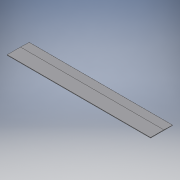
# Autodesk Inventor part: test_base
Saved by Autodesk Inventor 2018.1 (Build 221171000, 171)
## iProperties
Created: 2017-11-02
Part Number: test_base
Material: 一般
Document SubType Name: Modeling
Designer: kuwano
Density: 1 g/cm^3
Appearance: 既定
Author: kuwano
Autodesk Inventor part; units mm, degrees
ref_plane "XZ Plane" through (0, 0, 0) normal (0, 1, 0) x (-1, 0, 0)
sketch "スケッチ1" plane through (0, 0, 0) normal (1, 0, 0) x (0, 1, 0)
  line L0 (0, 120) -> (0, 0)
  line L1 (0, 0) -> (-3.0007, -80.0375)
  line L2 (-5, -80) -> (-5, 120)
  line L3 (-5, 120) -> (0, 120)
  arc A0 (-5, -80) -> (-3.0007, -80.0375) centre (-4, -80) ccw
  dimension "d0" = 120
  dimension "d1" = 1
  dimension "d2" = 5
  dimension "d3" = 80
  constraints: 8 end point, 2 point on circle, 2 tangent, 1 centre point, 1 parallel, 1 perpendicular, 1 vertical
  measures "d0" distance of L0.start L0.end
  measures "d1" radius of A0
  measures "d2" distance of L2.end L0.start
  measures "d3" vertical distance of A0.centre L0.end
ref_plane "作業平面1" through (650, 0, 0) normal (1, 0, 0) x (0, 1, 0)
sketch "スケッチ2" plane through (650, 0, 0) normal (1, 0, 0) x (0, 1, 0)
  line L0 (0, 120) -> (0, 0)
  line L1 (0, 0) -> (-3.0007, -80.0375)
  line L2 (-5, -80) -> (-5, 120)
  line L3 (-5, 120) -> (0, 120)
  arc A0 (-5, -80) -> (-3.0007, -80.0375) centre (-4, -80) ccw
  dimension "d5" = 120
  dimension "d6" = 1
  dimension "d7" = 5
  dimension "d8" = 80
  constraints: 8 end point, 2 point on circle, 2 tangent, 1 centre point, 1 parallel, 1 perpendicular, 1 vertical
  measures "d5" distance of L0.start L0.end
  measures "d6" radius of A0
  measures "d7" distance of L2.end L0.start
  measures "d8" vertical distance of A0.centre L0.end
ref_plane "作業平面2" through (-650, 0, 0) normal (1, 0, 0) x (0, 1, 0)
sketch "スケッチ3" plane through (-650, 0, 0) normal (1, 0, 0) x (0, 1, 0)
  line L0 (0, 120) -> (0, 0)
  line L1 (0, 0) -> (-3.0007, -80.0375)
  line L2 (-5, -80) -> (-5, 120)
  line L3 (-5, 120) -> (0, 120)
  arc A0 (-5, -80) -> (-3.0007, -80.0375) centre (-4, -80) ccw
  dimension "d10" = 120
  dimension "d11" = 1
  dimension "d12" = 5
  dimension "d13" = 80
  constraints: 8 end point, 2 point on circle, 2 tangent, 1 centre point, 1 parallel, 1 perpendicular, 1 vertical
  measures "d10" distance of L0.start L0.end
  measures "d11" radius of A0
  measures "d12" distance of L2.end L0.start
  measures "d13" vertical distance of A0.centre L0.end
loft "ロフト1" add profiles "スケッチ3", "スケッチ1", "スケッチ2"
